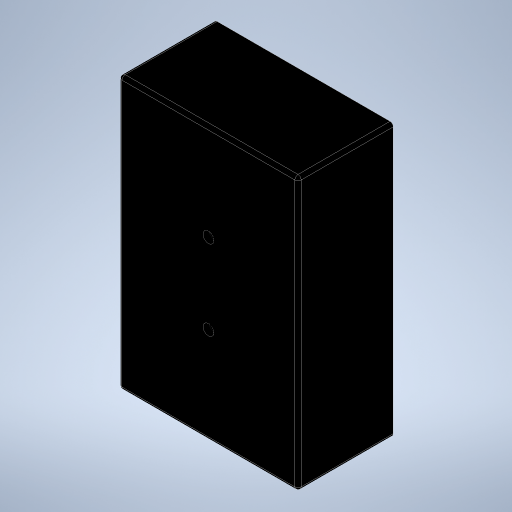
# Autodesk Inventor part: BatteryCase_Botton
Saved by Autodesk Inventor 2024 (Build 280153000, 153)
## iProperties
Created: 2023-12-27
Part Number: BatteryCase_Botton
Material: Generisch
Document SubType Name: Modeling
Designer: denni
Density: 1 g/cm^3
Appearance: Vorgabe(1)
Author: denni
Autodesk Inventor part; units mm, degrees
ref_plane "YZ Plane" through (0, 0, 0) normal (1, 0, 0) x (0, 1, 0)
ref_plane "XZ Plane" through (0, 0, 0) normal (0, 1, 0) x (-1, 0, 0)
ref_plane "XY Plane" through (0, 0, 0) normal (0, 0, 1) x (1, 0, 0)
sketch "Skizze1" plane through (0, 0, 0) normal (1, 0, 0) x (0, 1, 0)
  circle A0 centre (0, 0) radius 7.75
  line L0 (0, 0) -> (7.75, 0) construction
  circle A1 centre (17, 0) radius 7.75
  circle A2 centre (34, 0) radius 7.75
  circle A3 centre (51, 0) radius 7.75
  line L1 (66, 3.75) -> (-15, 3.75)
  line L2 (-15, 3.75) -> (-15, 9.75)
  line L3 (-15, 9.75) -> (66, 9.75)
  line L4 (66, 9.75) -> (66, 3.75)
  point P0 (24.75, 0)
  point P1 (41.75, 0)
  point P2 (58.75, 0)
  point P3 (66, 6.75)
  point P4 (-6.7823, 3.75)
  point P5 (6.7823, 3.75)
  point P6 (10.2177, 3.75)
  point P7 (23.7823, 3.75)
  point P8 (27.2177, 3.75)
  point P9 (40.7823, 3.75)
  point P10 (44.2177, 3.75)
  point P11 (57.7823, 3.75)
  dimension "d0" = 15.5
  dimension "d3" = 17
  dimension "a" = 9.75
  dimension "b" = 15
  dimension "d10" = 15
  dimension "d11" = 6
  constraints: 10 end point, 6 horizontal, 2 parallel, 1 coincident, 1 midpoint, 1 perpendicular, 18 other
  measures "d3" distance of L0.start point (17, 0)
  measures "a" distance from line of point (51, 0) L3
  measures "b" horizontal distance of point (66, 6.75) point (51, 0)
  measures "d10" distance from line of L2 point (0, 0)
  measures "d11" distance between parallel lines of L1 L3
extrude "Extrusion1" add sketch "Skizze1" along normal blind 10 contours A0 L1 L2 L3 L4 A3 A2 A1
sketch "Skizze2" plane through (0, -15, 9.75) normal (0, 0, 1) x (1, 0, 0)
  line L0 (0, 81) -> (10, 81) projected
  line L1 (10, 81) -> (-16, 81)
  line L2 (-16, 81) -> (-16, 0)
  line L3 (-16, 0) -> (10, 0)
  line L4 (10, 0) -> (10, 81)
  line L5 (0, 0) -> (10, 0) projected
  point P0 (0, 15)
  dimension "d14" = 26
  constraints: 8 end point, 2 parallel, 1 collinear, 1 horizontal, 1 perpendicular
  measures "d14" distance of L0.end L1.end
extrude "Extrusion2" add sketch "Skizze2" along normal blind 3
sketch "Skizze3" plane through (10, 0, 0) normal (1, 0, 0) x (0, 0, -1)
  line L0 (-12.75, 66) -> (-12.75, -15) projected
  line L1 (-12.75, 66) -> (17, 66)
  line L2 (17, 66) -> (17, -15)
  line L3 (17, -15) -> (-12.75, -15)
  line L4 (-12.75, -15) -> (-12.75, 66)
  line L5 (-3.75, -15) -> (-12.75, -15) construction
  circle A0 centre (17, 51) radius 2.5 construction
  point P0 (0, 0)
  point P1 (-12.75, -15)
  constraints: 8 end point, 2 parallel, 1 collinear, 1 horizontal, 1 perpendicular, 1 point on line
extrude "Extrusion3" add sketch "Skizze3" along normal blind 2
sketch "Skizze4" plane through (-16, -15, 9.75) normal (0, -1, 0) x (1, 0, 0)
  line L0 (0, 3) -> (28, 3) projected
  line L1 (28, -26.75) -> (28, 3) projected
  line L2 (0, 3) -> (28, 3)
  line L3 (28, 3) -> (28, -26.75)
  line L4 (28, -26.75) -> (0, -26.75)
  line L5 (0, -26.75) -> (0, 3)
  point P0 (16, -9.75)
  constraints: 8 end point, 2 parallel, 1 horizontal, 1 perpendicular
extrude "Extrusion4" add sketch "Skizze4" along normal blind 2
sketch "Skizze5" plane through (-16, 66, 9.75) normal (0, 1, 0) x (1, 0, 0)
  line L0 (0, 0) -> (0, 26.75) projected
  line L1 (28, -3) -> (0, -3)
  line L2 (0, -3) -> (0, 26.75)
  line L3 (0, 26.75) -> (28, 26.75)
  line L4 (28, 26.75) -> (28, -3)
  point P0 (16, 9.75)
  constraints: 8 end point, 2 parallel, 1 horizontal, 1 perpendicular
extrude "Extrusion5" add sketch "Skizze5" along normal blind 2
sketch "Skizze6" plane through (10, -15, -17) normal (0, 0, -1) x (-1, 0, 0)
  line L0 (-2, -2) -> (26, -2) projected
  line L1 (-2, -2) -> (4, -2)
  line L2 (4, -2) -> (4, 4)
  line L3 (4, 4) -> (-2, 4)
  line L4 (-2, 4) -> (-2, -2)
  line L5 (-2, 83) -> (26, 83) projected
  line L6 (-2, 83) -> (4, 83)
  line L7 (4, 83) -> (4, 77)
  line L8 (4, 77) -> (-2, 77)
  line L9 (-2, 77) -> (-2, 83)
  point P0 (10, 15)
  point P1 (4, 83)
  dimension "d23" = 6
  constraints: 16 end point, 4 parallel, 3 equal length, 2 horizontal, 2 perpendicular
  measures "d23" distance of L1.end L2.end
extrude "Extrusion6" add sketch "Skizze6" against normal up to surface (20.75 mm away)
fillet "Rundung1" radius 1 8 edges at (10, -11, -6.625) (6, -11, -6.625) (6, -15, -6.625) (12, -17, -2.125) (12, 68, -2.125) (10, 62, -6.625) (6, 62, -6.625) (6, 66, -6.625)
sketch "Skizze8" plane through (5, 66, -17) normal (0, 0, -1) x (-1, 0, 0)
  arc A0 (-6, 2) -> (-7, 1) centre (-6, 1) ccw construction
  arc A1 (-2, -4) -> (-1, -3) centre (-2, -3) ccw construction
  line L0 (-6, 1) -> (-2, -3) construction
  arc A2 (-7, -82) -> (-6, -83) centre (-6, -82) ccw construction
  line L1 (-6, -82) -> (-2, -78) construction
  point P0 (5, -66)
  point P1 (-4, -80)
  point P2 (-4, -1)
  constraints: 4 end point, 2 midpoint
hole "Bohrung1" at (9, -14, -17) at (9, 65, -17) direction (0, 0, 1) diameter 3.2 depth 3
hole "Bohrung2" at (9, 65, -17) at (9, -14, -17) direction (0, 0, 1) diameter 2.4 depth 15 clearance for "Inbusschraube ISO 4762" size "M2" standard "ISO"
mirror "Spiegeln1" about plane through (-16, 66, 9.75) normal (-1, 0, 0) of "Extrusion1", "Extrusion2", "Extrusion3", "Extrusion4", "Extrusion5", "Extrusion6", "Rundung1", "Bohrung1", "Bohrung2"
sketch "Skizze7" plane through (0, -15, 9.75) normal (0, 0, -1) x (-1, 0, 0)
  line L0 (0, 81) -> (0, 0) projected
  line L1 (32, 0) -> (0, 0) projected
  line L2 (32, 81) -> (32, 0) projected
  line L3 (0, 81) -> (32, 81) projected
  point P0 (0, 15)
extrude "Extrusion7" add sketch "Skizze7" along normal blind 1
fillet "Rundung2" radius 1 8 edges at (-43.7071, 67.7071, 12.75) (-44, 25.5, 12.75) (-43.7071, -16.7071, 12.75) (-16, -17, 12.75) (11.7071, -16.7071, 12.75) (12, 25.5, 12.75) (11.7071, 67.7071, 12.75) (-16, 68, 12.75)
sketch "Skizze9" plane through (0, -15, 8.75) normal (0, 0, -1) x (-1, 0, 0)
  line L0 (0, 81) -> (32, 81) construction
  line L1 (16, 81) -> (16, 53) construction
  line L2 (16, 53) -> (16, 28) construction
  line L3 (16, 28) -> (16, 0) construction
  line L4 (32, 0) -> (0, 0) construction
  point P0 (0, 15)
  dimension "d44" = 25
  constraints: 6 end point, 2 coincident, 2 collinear, 2 midpoint, 1 vertical
  measures "d44" distance of L1.end L2.end
hole "Bohrung3" at (-16, 38, 8.75) at (-16, 13, 8.75) direction (0, 0, 1) diameter 3.4 end through all countersink diameter 7.5 countersink angle 90 clearance for "Innensechskant-Senkkopfschraube ISO 10642" size "M3" standard "ISO"
equation "\"d10\" = b"
